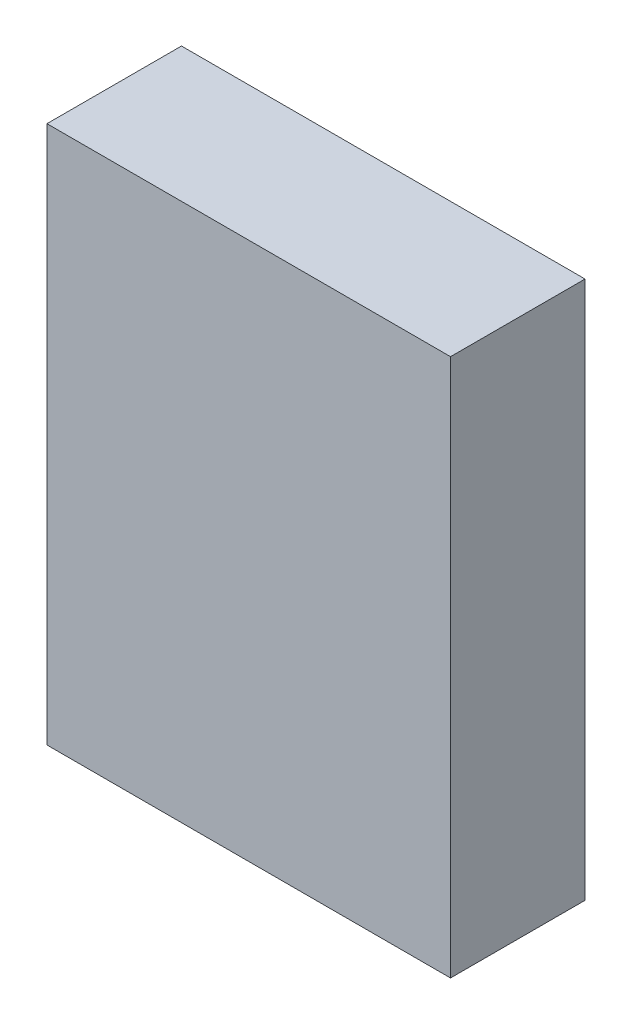
# Autodesk Inventor part: dummy box
Saved by Autodesk Inventor 2024.2 (Build 282272000, 272)
## iProperties
Created: 2024-03-15
Part Number: dummy box
Material: Generic
Document SubType Name: Modeling
Designer: admin
Density: 1 g/cm^3
Appearance: Default
Author: admin
Autodesk Inventor part; units mm, degrees
ref_plane "YZ Plane" through (0, 0, 0) normal (1, 0, 0) x (0, 1, 0)
ref_plane "XZ Plane" through (0, 0, 0) normal (0, 1, 0) x (-1, 0, 0)
ref_plane "XY Plane" through (0, 0, 0) normal (0, 0, 1) x (1, 0, 0)
sketch "Sketch1" plane through (0, 0, 0) normal (0, 0, 1) x (1, 0, 0)
  line L0 (-300, 400) -> (300, 400)
  line L1 (300, 400) -> (300, -400)
  line L2 (300, -400) -> (-300, -400)
  line L3 (-300, -400) -> (-300, 400)
  line L4 (-300, 400) -> (300, -400) construction
  line L5 (300, 400) -> (-300, -400) construction
  point P0 (0, 0)
  dimension "d0" = 600
  dimension "d1" = 800
  constraints: 12 end point, 2 midpoint, 2 parallel, 1 horizontal, 1 perpendicular
  measures "d0" distance of L1.end L2.end
  measures "d1" distance of L0.end L1.end
extrude "Extrusion1" add sketch "Sketch1" along normal blind 200
body "Solid1"
